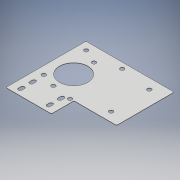
# Autodesk Inventor part: pieza2
Saved by Autodesk Inventor 2018 (Build 220112000, 112)
## iProperties
Created: 2018-10-05
Part Number: pieza2
Material: Genérico
Document SubType Name: Modeling
Designer: Vayron
Density: 1 g/cm^3
Appearance: Valor por defecto
Author: Vayron
Autodesk Inventor part; units mm, degrees
ref_plane "YZ Plane" through (0, 0, 0) normal (1, 0, 0) x (0, 1, 0)
ref_plane "XZ Plane" through (0, 0, 0) normal (0, 1, 0) x (-1, 0, 0)
ref_plane "XY Plane" through (0, 0, 0) normal (0, 0, 1) x (1, 0, 0)
sketch "Boceto1" plane through (0, 0, 0) normal (0, 0, 1) x (1, 0, 0)
  line L0 (98.53, 89.5715) -> (-98.53, 89.5715)
  line L1 (-98.53, -89.5715) -> (98.53, 89.5715) construction
  line L2 (98.53, -89.5715) -> (-98.53, 89.5715) construction
  line L3 (3.26, -89.5715) -> (3.26, -39.0815)
  line L4 (3.26, -39.0815) -> (98.53, -39.0815)
  line L5 (98.53, 89.5715) -> (98.53, -39.0815)
  circle A0 centre (65.96, 66.7715) radius 4.5
  circle A1 centre (65.96, -18.7285) radius 4.5
  circle A2 centre (-80.61, 72.0615) radius 4.5
  circle A3 centre (-4.48, 76.5415) radius 4.5
  circle A4 centre (-80.61, -22.7985) radius 4.5
  circle A5 centre (-4.48, -40.0285) radius 4.5
  circle A6 centre (-48.45, -33.5185) radius 4.5
  circle A7 centre (-48.45, 57.2715) radius 4.5
  circle A8 centre (-48.45, 11.8765) radius 31.755
  line L6 (-83.4615, -46.0315) -> (-83.4615, -51.6915)
  line L7 (-75.3185, -51.6915) -> (-75.3185, -46.0315)
  line L8 (-83.4615, -76.9315) -> (-83.4615, -71.2715)
  line L9 (-75.3185, -71.2715) -> (-75.3185, -76.9315)
  arc A9 (-75.3185, -46.0315) -> (-83.4615, -46.0315) centre (-79.39, -46.0315) ccw
  arc A10 (-83.4615, -51.6915) -> (-75.3185, -51.6915) centre (-79.39, -51.6915) ccw
  arc A11 (-75.3185, -71.2715) -> (-83.4615, -71.2715) centre (-79.39, -71.2715) ccw
  arc A12 (-83.4615, -76.9315) -> (-75.3185, -76.9315) centre (-79.39, -76.9315) ccw
  line L10 (-19.9515, -46.0315) -> (-19.9515, -51.6915)
  line L11 (-11.8085, -51.6915) -> (-11.8085, -46.0315)
  line L12 (-19.9515, -71.2715) -> (-19.9515, -76.9315)
  line L13 (-11.8085, -71.2715) -> (-11.8085, -76.9315)
  arc A13 (-11.8085, -46.0315) -> (-19.9515, -46.0315) centre (-15.88, -46.0315) ccw
  arc A14 (-19.9515, -51.6915) -> (-11.8085, -51.6915) centre (-15.88, -51.6915) ccw
  arc A15 (-11.8085, -71.2715) -> (-19.9515, -71.2715) centre (-15.88, -71.2715) ccw
  arc A16 (-19.9515, -76.9315) -> (-11.8085, -76.9315) centre (-15.88, -76.9315) ccw
  line L14 (-98.53, 89.5715) -> (-98.53, -89.5715)
  line L15 (-98.53, -89.5715) -> (3.26, -89.5715)
  point P0 (0, 0)
  dimension "d6" = 9
  dimension "d8" = 9
  dimension "d13" = 9
  dimension "d14" = 9
  dimension "d18" = 9
  dimension "d19" = 9
  dimension "d22" = 9
  dimension "d24" = 9
  dimension "d26" = 63.51
  constraints: 32 end point, 17 centre point, 16 point on circle, 8 tangent, 6 vertical, 3 parallel, 2 midpoint, 1 horizontal
  measures "d6" diameter of A0
  measures "d8" diameter of A1
  measures "d13" diameter of A2
  measures "d14" diameter of A3
  measures "d18" diameter of A4
  measures "d19" diameter of A5
  measures "d22" diameter of A6
  measures "d24" diameter of A7
  measures "d26" diameter of A8
extrude "Extrusión1" add sketch "Boceto1" along normal mid plane 0.8
fillet "Empalme1" radius 3 6 edges at (98.53, 89.5715, 0) (98.53, -39.0815, 0) (3.26, -89.5715, 0) (3.26, -39.0815, 0) (-98.53, -89.5715, 0) (-98.53, 89.5715, 0)
